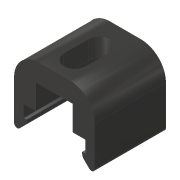
# Autodesk Inventor part: IR_Focus_Dark
Saved by Autodesk Inventor 2019 (Build 230136000, 136)
## iProperties
Created: 2023-04-01
Part Number: IR_Focus_Dark
Material: Generic
Document SubType Name: Modeling
Designer: Oudenas
Density: 1 g/cm^3
Appearance: Default
Author: Oudenas
Autodesk Inventor part; units mm, degrees
ref_plane "YZ Plane" through (0, 0, 0) normal (1, 0, 0) x (0, 1, 0)
ref_plane "XZ Plane" through (0, 0, 0) normal (0, 1, 0) x (-1, 0, 0)
ref_plane "XY Plane" through (0, 0, 0) normal (0, 0, 1) x (1, 0, 0)
sketch "Sketch1" plane through (0, 0, 0) normal (0, 1, 0) x (-1, 0, 0)
  line L0 (6.5, 5.75) -> (-6.5, 5.75)
  line L1 (-6.5, 5.75) -> (-6.5, -5.75)
  line L2 (-6.5, -5.75) -> (6.5, -5.75)
  line L3 (6.5, -5.75) -> (6.5, 5.75)
  line L4 (6.5, 5.75) -> (-6.5, -5.75) construction
  line L5 (-6.5, 5.75) -> (6.5, -5.75) construction
  point P0 (0, 0)
  dimension "d0" = 13
  dimension "d1" = 11.5
  constraints: 12 end point, 2 midpoint, 2 parallel, 1 horizontal, 1 perpendicular
  measures "d0" distance of L2.end L1.end
  measures "d1" distance of L1.end L0.end
extrude "Extrusion1" add sketch "Sketch1" along normal blind 7
sketch "Sketch2" plane through (0, 0, 0) normal (0, -1, 0) x (1, 0, 0)
  line L0 (3, 5.75) -> (-3, 5.75)
  line L1 (-3, 5.75) -> (-3, -4.75)
  line L2 (-3, -4.75) -> (3, -4.75)
  line L3 (3, -4.75) -> (3, 5.75)
  line L4 (3, 5.75) -> (-3, -4.75) construction
  line L5 (-3, 5.75) -> (3, -4.75) construction
  line L6 (-6.5, 5.75) -> (6.5, 5.75) projected
  point P0 (0, 0)
  point P1 (0, 0.5)
  dimension "d4" = 6
  dimension "d5" = 10.5
  constraints: 12 end point, 2 midpoint, 2 parallel, 1 collinear, 1 horizontal, 1 perpendicular
  measures "d4" distance of L2.end L1.end
  measures "d5" distance of L1.end L0.end
extrude "Extrusion2" cut sketch "Sketch2" against normal blind 4
sketch "Sketch4" plane through (0, 4, 0) normal (0, -1, 0) x (1, 0, 0)
  line L0 (0, 4.25) -> (0, -3.35) construction
  line L1 (-1.8, 2.45) -> (-1.8, -1.55)
  line L2 (1.8, -1.55) -> (1.8, 2.45)
  arc A0 (1.8, 2.45) -> (-1.8, 2.45) centre (0, 2.45) ccw
  arc A1 (-1.8, -1.55) -> (1.8, -1.55) centre (0, -1.55) ccw
  line L3 (-3, 5.75) -> (3, 5.75) projected
  point P0 (0, 0)
  point P1 (0, 0.45)
  dimension "d15" = 3.6
  dimension "d16" = 4
  dimension "d17" = 3.3
  constraints: 8 end point, 6 point on circle, 4 tangent, 2 centre point, 2 point on line, 1 midpoint, 1 parallel, 1 vertical
  measures "d15" diameter of A1
  measures "d16" distance of A0.centre A1.centre
  measures "d17" distance from line of A0.centre L3
extrude "Extrusion4" cut sketch "Sketch4" against normal blind 3
sketch "Sketch5" plane through (0, 0, 0) normal (0, -1, 0) x (1, 0, 0)
  line L0 (6.5, 5.75) -> (6.5, -5.75) projected
  line L1 (3, 5.75) -> (6.5, 5.75) projected
  line L2 (6.5, -5.75) -> (5, -5.75)
  line L3 (5, -5.75) -> (5, 5.75)
  line L4 (5, 5.75) -> (6.5, 5.75)
  line L5 (6.5, 5.75) -> (6.5, -5.75)
  line L6 (-6.5, -5.75) -> (-6.5, 5.75) projected
  line L7 (-6.5, 5.75) -> (-3, 5.75) projected
  line L8 (-6.5, -5.75) -> (-5, -5.75)
  line L9 (-5, -5.75) -> (-5, 5.75)
  line L10 (-5, 5.75) -> (-6.5, 5.75)
  line L11 (-6.5, 5.75) -> (-6.5, -5.75)
  point P0 (0, 0)
  dimension "d24" = 1.5
  dimension "d25" = 1.5
  constraints: 16 end point, 4 parallel, 2 horizontal, 2 perpendicular, 2 point on line
  measures "d24" distance of L3.end L4.end
  measures "d25" distance of L10.end L9.end
extrude "Extrusion5" add sketch "Sketch5" along normal blind 2
sketch "Sketch6" plane through (0, -2, 0) normal (0, -1, 0) x (1, 0, 0)
  line L0 (6.5, 5.75) -> (6.5, -5.75) projected
  line L1 (6.5, -5.75) -> (4.5, -5.75)
  line L2 (4.5, -5.75) -> (4.5, 5.75)
  line L3 (4.5, 5.75) -> (6.5, 5.75)
  line L4 (6.5, 5.75) -> (6.5, -5.75)
  line L5 (-6.5, -5.75) -> (-6.5, 5.75) projected
  line L6 (-6.5, -5.75) -> (-4.5, -5.75)
  line L7 (-4.5, -5.75) -> (-4.5, 5.75)
  line L8 (-4.5, 5.75) -> (-6.5, 5.75)
  line L9 (-6.5, 5.75) -> (-6.5, -5.75)
  point P0 (0, 0)
  dimension "d28" = 2
  dimension "d29" = 2
  constraints: 16 end point, 4 parallel, 2 horizontal, 2 perpendicular, 1 point on line
  measures "d28" distance of L2.end L3.end
  measures "d29" distance of L8.end L7.end
extrude "Extrusion6" add sketch "Sketch6" along normal blind 2
chamfer "Chamfer2" distance 1.4 angle 45 2 edges at (4.5, -4, 0) (-4.5, -4, 0)
fillet "Fillet2" radius 1 2 edges at (4.5, -2.6, 0) (-4.5, -2.6, 0)
fillet "Fillet3" radius 0.5 4 edges at (6.5, -4, 0) (5.9, -4, 0) (-6.5, -4, 0) (-5.9, -4, 0)
fillet "Fillet4" radius 4 2 edges at (6.5, 7, 0) (-6.5, 7, 0)
body "Solid1"
